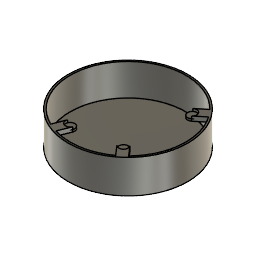
OutShellBase2_v3 (Autodesk Fusion 360 design; units mm, degrees)
Autodesk Fusion 360 part; units mm, degrees
sketch "Sketch1" plane through (0, 0, 0) normal (0, 0, 1) x (1, 0, 0)
  circle A0 centre (0, 0) radius 66
  dimension "d1" = 132
  constraint coincident A0.centre origin
  measures "d1" diameter of A0
extrude "Extrude1" add sketch "Sketch1" against normal blind 37
shell "Shell1" thickness 2 removed faces 1 at (19.2692, 15.933, 0)
sketch "Sketch3" plane through (0, 0, 0) normal (0, 0, 1) x (-1, 0, 0)
  circle A0 centre (-38.9288, -32.0709) radius 5.1
  circle A1 centre (-32.7653, 37.8108) radius 5.1
  circle A2 centre (18, 46) radius 5.1
  circle A3 centre (0, 0) radius 64
  circle A4 centre (0, 0) radius 66
  line L0 (22.7493, 44.1416) -> (13.2507, 47.8584) construction
  line L1 (-36.6195, 34.4709) -> (-28.9111, 41.1507) construction
  line L2 (-35.6859, -36.0071) -> (-42.1716, -28.1346) construction
  line L3 (-35.6859, -36.0071) -> (-45.9962, -44.5012)
  line L4 (-42.1716, -28.1346) -> (-52.4818, -36.6287)
  line L5 (-45.9962, -44.5012) -> (-52.4818, -36.6287) construction
  line L6 (-28.9111, 41.1507) -> (-37.9251, 51.5528)
  line L7 (-36.6195, 34.4709) -> (-45.6335, 44.873)
  line L8 (-37.9251, 51.5528) -> (-45.6335, 44.873) construction
  line L9 (22.7493, 44.1416) -> (27.9967, 57.5516)
  line L10 (13.2507, 47.8584) -> (18.4981, 61.2684)
  line L11 (27.9967, 57.5516) -> (18.4981, 61.2684) construction
  point P0 (18, 46)
  point P1 (-32.7653, 37.8108)
  point P2 (-38.9288, -32.0709)
  dimension "d5" = 10.2
  dimension "d6" = 10.2
  dimension "d7" = 10.2
  constraint midpoint L0 P0
  constraint coincident P0 A2.centre
  constraint coincident A2 L0.end
  constraint midpoint L1 P1
  constraint coincident P1 A1.centre
  constraint coincident A1 L1.end
  constraint midpoint L2 P2
  constraint coincident P2 A0.centre
  constraint coincident A0 L2.end
  constraint coincident A3 L3.end
  constraint coincident A3 L4.end
  constraint parallel L3 L4
  constraint tangent A0 L3
  constraint parallel L2 L5
  constraint coincident A3 L6.end
  constraint tangent A1 L6
  constraint coincident A3 L7.end
  constraint tangent A1 L7
  constraint perpendicular L1 L7
  constraint parallel L1 L8
  constraint coincident A3 L9.end
  constraint tangent A2 L9
  constraint perpendicular L0 L9
  constraint coincident A3 L10.end
  constraint tangent A2 L10
  constraint parallel L0 L11
  measures "d5" diameter of A0
  measures "d6" diameter of A1
extrude "Extrude2" add sketch "Sketch3" against normal blind 5 contours A0 | A0 A3 L3 L4 | A1 A3 L6 L7 | A1 | A2 A3 L9 L10 | A2
extrude "Extrude3" cut sketch "Sketch3" against normal blind 2.75 contours A0 | A1 | A2
equation "d1 = ( 66 * 2 ) * 1 mm"
